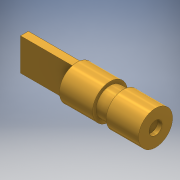
# Autodesk Inventor part: laser_realpoo_4mm
Saved by Autodesk Inventor 2016 (Build 200138000, 138)
## iProperties
Created: 2016-08-08
Part Number: laser_realpoo_4mm
Material: Brass, Soft Yellow
Document SubType Name: Modeling
Designer: rawrdong
Density: 8.47 g/cm^3
Appearance: Brass - Satin
Author: rawrdong
Autodesk Inventor part; units mm, degrees
ref_plane "YZ Plane" through (0, 0, 0) normal (1, 0, 0) x (0, 1, 0)
ref_plane "XZ Plane" through (0, 0, 0) normal (0, 1, 0) x (-1, 0, 0)
ref_plane "XY Plane" through (0, 0, 0) normal (0, 0, 1) x (1, 0, 0)
sketch "Sketch1" plane through (0, 0, 0) normal (0, 0, 1) x (1, 0, 0)
  line L0 (0, 0) -> (9.0087, 0)
  line L1 (0, 0) -> (0, 2)
  line L2 (0, 2) -> (3.8, 2)
  line L3 (3.8, 2) -> (3.8, 1.6)
  line L4 (3.8, 1.6) -> (5.3087, 1.6)
  line L5 (5.3087, 1.6) -> (5.3087, 1.95)
  line L6 (5.3087, 1.95) -> (9.0087, 1.95)
  line L7 (9.0087, 1.95) -> (9.0087, 0.75)
  line L8 (9.0087, 0.75) -> (8.5087, 0.75)
  line L9 (8.5087, 0.75) -> (8.5087, 0)
  dimension "d0" = 4
  dimension "d1" = 3.9
  dimension "d2" = 3.8
  dimension "d3" = 3.7
  dimension "d5" = 3.2
  dimension "d10" = 1.5
  dimension "d11" = 0.5
  constraints: 21 end point, 6 perpendicular, 2 horizontal, 1 point on line, 1 vertical
  measures "d0" diameter of L2 L0
  measures "d1" diameter of L6 L0
  measures "d2" distance of L1.end L2.end
  measures "d3" distance of L5.end L6.end
  measures "d5" diameter of L4 L0
  measures "d10" diameter of L8 L0
  measures "d11" distance of L7.end L8.end
revolve "Revolution1" add sketch "Sketch1" angle 360 about axis through (0, 0, 0) along (1, 0, 0)
sketch "Sketch2" plane through (0, 0, 0) normal (-1, 0, 0) x (0, 0, 1)
  line L0 (-1.85, -0.45) -> (1.85, -0.45)
  line L1 (1.85, -0.45) -> (1.85, 0.45)
  line L2 (1.85, 0.45) -> (-1.85, 0.45)
  line L3 (-1.85, 0.45) -> (-1.85, -0.45)
  line L4 (-1.85, -0.45) -> (1.85, 0.45) construction
  line L5 (1.85, -0.45) -> (-1.85, 0.45) construction
  point P0 (0, 0)
  dimension "d6" = 3.7
  dimension "d7" = 0.9
  constraints: 12 end point, 2 midpoint, 2 parallel, 1 horizontal, 1 perpendicular
  measures "d6" distance of L0.start L0.end
  measures "d7" distance of L0.end L1.end
extrude "Extrusion1" add sketch "Sketch2" along normal blind 6
body "Solid1"
